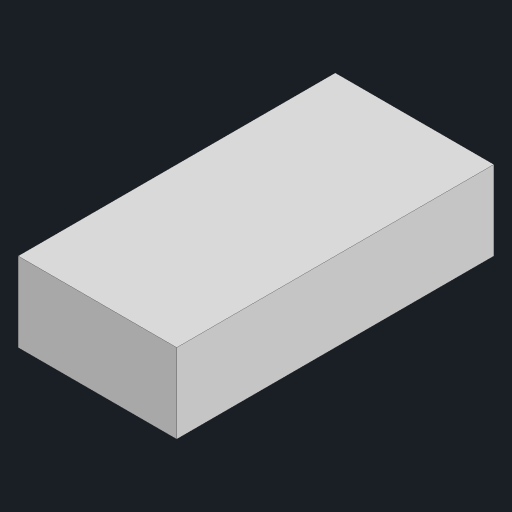
# Autodesk Inventor part: Styrofoam
Saved by Autodesk Inventor 2023.1 (Build 271208000, 208)
## iProperties
Created: 2022-11-03
Part Number: Styrofoam
Material: Generic
Document SubType Name: Modeling
Designer: Jarrett
Density: 1 g/cm^3
Appearance: Default
Author: Jarrett
Autodesk Inventor part; units mm, degrees
ref_plane "YZ Plane" through (0, 0, 0) normal (1, 0, 0) x (0, 1, 0)
ref_plane "XZ Plane" through (0, 0, 0) normal (0, 1, 0) x (-1, 0, 0)
ref_plane "XY Plane" through (0, 0, 0) normal (0, 0, 1) x (1, 0, 0)
sketch "Sketch1" plane through (0, 0, 0) normal (0, 1, 0) x (-1, 0, 0)
  line L0 (-50.8, 101.6) -> (50.8, 101.6)
  line L1 (50.8, 101.6) -> (50.8, -101.6)
  line L2 (50.8, -101.6) -> (-50.8, -101.6)
  line L3 (-50.8, -101.6) -> (-50.8, 101.6)
  line L4 (-50.8, 101.6) -> (50.8, -101.6) construction
  line L5 (50.8, 101.6) -> (-50.8, -101.6) construction
  point P0 (0, 0)
  dimension "d0" = 101.6
  dimension "d1" = 203.2
  constraints: 12 end point, 2 midpoint, 2 parallel, 1 horizontal, 1 perpendicular
  measures "d0" distance of L1.end L2.end
  measures "d1" distance of L0.end L1.end
extrude "Extrusion1" add sketch "Sketch1" along normal blind 50.8
body "Solid1"
